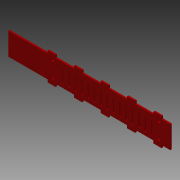
# Autodesk Inventor part: SidePanel_Rail_v2_diag
Saved by Autodesk Inventor 2015 SP1 (Build 190203100, 203)
## iProperties
Created: 2014-08-06
Part Number: SidePanel_Rail_v2_diag
Material: Acrylic
Document SubType Name: Modeling
Designer: Patrick Camilleri
Density: 1.188 g/cm^3
Appearance: Smooth - Red
Author: Patrick Camilleri
Autodesk Inventor part; units mm, degrees
ref_plane "YZ Plane" through (0, 0, 0) normal (1, 0, 0) x (0, 1, 0)
ref_plane "XZ Plane" through (0, 0, 0) normal (0, 1, 0) x (-1, 0, 0)
ref_plane "XY Plane" through (0, 0, 0) normal (0, 0, 1) x (1, 0, 0)
sketch "Sketch1" plane through (0, 0, 0) normal (0, 1, 0) x (-1, 0, 0)
  line L0 (21.065, 194.93) -> (-21.065, 194.93)
  line L1 (-21.065, 194.93) -> (-21.065, -110.93)
  line L2 (-21.065, -110.93) -> (21.065, -110.93)
  line L3 (21.065, -110.93) -> (21.065, 194.93)
  line L4 (21.065, 0) -> (-21.065, 0) construction
  line L5 (0, -110.93) -> (0, 194.93) construction
  point P0 (0, 0)
  point P1 (0, 0)
  dimension "d57" = 42.13
  dimension "d58" = 110.93
  dimension "d59" = 194.93
  constraints: 12 end point, 3 midpoint, 2 parallel, 2 perpendicular, 2 point on line, 1 coincident, 1 horizontal
  measures "d57" distance of L1.end L2.end
  measures "d58" distance between parallel lines of L4 L2
  measures "d59" distance between parallel lines of L4 L0
extrude "Extrusion1" add sketch "Sketch1" along normal blind 3
sketch "Sketch3" plane through (0, 0, 0) normal (0, -1, 0) x (1, 0, 0)
  line L0 (21.065, -110.93) -> (-21.065, -110.93) projected
  line L1 (21.065, 194.93) -> (21.065, -110.93) projected
  line L2 (-21.065, -110.93) -> (-21.065, 194.93) projected
  line L3 (-26.065, -79.365) -> (-21.065, -79.365)
  line L4 (-21.065, -79.365) -> (-21.065, -94.495)
  line L5 (-21.065, -94.495) -> (-26.065, -94.495)
  line L6 (-26.065, -94.495) -> (-26.065, -79.365)
  line L7 (-26.065, -79.365) -> (-21.065, -94.495) construction
  line L8 (-21.065, -79.365) -> (-26.065, -94.495) construction
  line L9 (26.065, -94.495) -> (21.065, -94.495)
  line L10 (21.065, -94.495) -> (21.065, -79.365)
  line L11 (21.065, -79.365) -> (26.065, -79.365)
  line L12 (26.065, -79.365) -> (26.065, -94.495)
  line L13 (26.065, -94.495) -> (21.065, -79.365) construction
  line L14 (21.065, -94.495) -> (26.065, -79.365) construction
  point P0 (0, 0)
  point P1 (-23.565, -86.93)
  point P2 (23.565, -86.93)
  point P3 (21.065, -86.93)
  dimension "d61" = 15.13
  dimension "d64" = 5
  dimension "d65" = 15.13
  dimension "d78" = 24
  dimension "d79" = 24
  dimension "d97" = 5
  constraints: 24 end point, 5 midpoint, 4 parallel, 2 horizontal, 2 perpendicular, 2 point on line
  measures "d61" distance of L3.end L4.end
  measures "d64" distance of L10.end L11.end
  measures "d65" distance of L9.end L10.end
  measures "d78" distance from line of L0 point (-23.565, -86.93)
  measures "d79" distance from line of L0 point (23.565, -86.93)
  measures "d97" distance between parallel lines of L6 L4
extrude "Extrusion3" add sketch "Sketch3" against normal blind 3
pattern_linear "Rectangular Pattern1" count 5 spacing 50 along (0, 0, 1) of "Extrusion3"
sketch "Sketch10" plane through (0, 3, 0) normal (0, 1, 0) x (1, 0, 0)
  line L0 (21.065, 110.93) -> (-21.065, 110.93) projected
  line L1 (-9.7, 74.43) -> (13.7, 74.43)
  line L2 (14.5, 75.23) -> (14.5, 76.63)
  line L3 (13.7, 77.43) -> (-9.7, 77.43)
  line L4 (-10.5, 76.63) -> (-10.5, 75.23)
  line L5 (-10.5, 74.43) -> (14.5, 77.43) construction
  line L6 (14.5, 74.43) -> (-10.5, 77.43) construction
  line L7 (-10.5, 74.43) -> (12.9, 74.43) construction
  arc A0 (-10.5, 75.23) -> (-9.7, 74.43) centre (-9.7, 75.23) ccw
  arc A1 (-9.7, 77.43) -> (-10.5, 76.63) centre (-9.7, 76.63) ccw
  arc A2 (13.7, 74.43) -> (14.5, 75.23) centre (13.7, 75.23) ccw
  arc A3 (14.5, 76.63) -> (13.7, 77.43) centre (13.7, 76.63) ccw
  point P0 (0, 0)
  point P1 (2, 75.93)
  point P2 (2, 75.93)
  dimension "d176" = 25
  dimension "d177" = 0
  dimension "d178" = 3
  dimension "d179" = 35
  dimension "d180" = 2
  dimension "d185" = 0.8
  constraints: 14 end point, 8 point on circle, 8 point on line, 8 tangent, 4 centre point, 3 equal radius, 3 midpoint, 2 parallel, 1 collinear, 1 horizontal, 1 perpendicular
  measures "d176" distance of L5.start L6.start
  measures "d177" distance between parallel lines of L7 L1
  measures "d178" distance of L5.end L6.start
  measures "d179" distance from line of L0 point (2, 75.93)
  measures "d180" horizontal distance of point (0, 0) point (2, 75.93)
  measures "d185" radius of A0
extrude "Extrusion7" cut sketch "Sketch10" against normal blind 10
sketch "Sketch11" plane through (0, 3, 0) normal (0, 1, 0) x (1, 0, 0)
  line L0 (21.065, 110.93) -> (-21.065, 110.93) projected
  line L1 (-21.065, 110.93) -> (-21.065, 94.495) projected
  line L2 (21.065, 94.495) -> (21.065, 110.93) projected
  line L3 (-15.935, 86.445) -> (-13.065, 86.445)
  line L4 (-13.065, 86.445) -> (-13.065, 91.415)
  line L5 (-13.065, 91.415) -> (-15.935, 91.415)
  line L6 (-15.935, 91.415) -> (-15.935, 86.445)
  line L7 (-15.935, 86.445) -> (-13.065, 91.415) construction
  line L8 (-13.065, 86.445) -> (-15.935, 91.415) construction
  line L9 (13.065, 86.445) -> (15.935, 86.445)
  line L10 (15.935, 86.445) -> (15.935, 91.415)
  line L11 (15.935, 91.415) -> (13.065, 91.415)
  line L12 (13.065, 91.415) -> (13.065, 86.445)
  line L13 (13.065, 86.445) -> (15.935, 91.415) construction
  line L14 (15.935, 86.445) -> (13.065, 91.415) construction
  point P0 (0, 0)
  point P1 (-14.5, 88.93)
  point P2 (14.5, 88.93)
  dimension "d136" = 2.87
  dimension "d137" = 4.97
  dimension "d140" = 22
  dimension "d186" = 14.5
  dimension "d187" = 14.5
  constraints: 24 end point, 4 midpoint, 4 parallel, 2 equal length, 2 horizontal, 2 perpendicular, 1 point on line
  measures "d136" distance of L5.end L4.end
  measures "d137" distance of L4.end L3.end
  measures "d140" distance from line of L0 point (-14.5, 88.93)
  measures "d186" horizontal distance of point (0, 0) point (-14.5, 88.93)
  measures "d187" horizontal distance of point (0, 0) point (14.5, 88.93)
extrude "Extrusion8" cut sketch "Sketch11" against normal blind 10
pattern_linear "Rectangular Pattern7" count 2 spacing 200 along (0, 0, 1) of "Extrusion8"
pattern_linear "Rectangular Pattern6" count 15 spacing 12 along (0, 0, 1) of "Extrusion7"
equation "\"d79\" = d78"
equation "\"kerf\" = 0.13"
equation "\"tab_w\" = 15"
equation "\"tab_h\" = 5"
body "Solid1"
